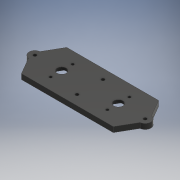
# Autodesk Inventor part: AC09
Saved by Autodesk Inventor 2017 (Build 210142000, 142)
## iProperties
Created: 2019-11-01
Part Number: AC09
Material: ABS Plastic
Document SubType Name: Modeling
Designer: Dell
Density: 1.06 g/cm^3
Appearance: Smooth - Black
Author: Dell
Autodesk Inventor part; units mm, degrees
ref_plane "YZ Plane" through (0, 0, 0) normal (1, 0, 0) x (0, 1, 0)
ref_plane "XZ Plane" through (0, 0, 0) normal (0, 1, 0) x (-1, 0, 0)
ref_plane "XY Plane" through (0, 0, 0) normal (0, 0, 1) x (1, 0, 0)
sketch "Sketch1" plane through (0, 0, 0) normal (0, 0, 1) x (1, 0, 0)
  circle A0 centre (0, 0) radius 3.5
  circle A1 centre (43.8036, 0) radius 3.5
  line L0 (-20.2073, 0) -> (-10.1036, 17.5)
  line L1 (-10.1036, 17.5) -> (10.1036, 17.5)
  line L2 (10.1036, 17.5) -> (20.2073, 0)
  line L3 (20.2073, 0) -> (10.1036, -17.5)
  line L4 (10.1036, -17.5) -> (-10.1036, -17.5)
  line L5 (-10.1036, -17.5) -> (-20.2073, 0)
  line L6 (64.0108, 0) -> (53.9072, -17.5)
  line L7 (53.9072, -17.5) -> (33.6999, -17.5)
  line L8 (33.6999, -17.5) -> (23.5963, 0)
  line L9 (23.5963, 0) -> (33.6999, 17.5)
  line L10 (33.6999, 17.5) -> (53.9072, 17.5)
  line L11 (53.9072, 17.5) -> (64.0108, 0)
  line L12 (10.1036, 17.5) -> (33.6999, 17.5)
  line L13 (10.1036, -17.5) -> (33.6999, -17.5)
  dimension "d0" = 7
  dimension "d1" = 7
  dimension "d2" = 43.8036
  dimension "d3" = 35
  constraints: 28 end point, 4 horizontal alignment, 3 coincident, 2 centre point, 2 horizontal, 26 other
  measures "d0" diameter of A0
  measures "d1" diameter of A1
  measures "d2" distance of A1.centre point (0, 0)
  measures "d3" distance between parallel lines of L4 L1
extrude "Extrusion1" add sketch "Sketch1" along normal blind 4
sketch "Sketch2" plane through (0, 0, 4) normal (0, 0, 1) x (1, 0, 0)
  circle A0 centre (43.8036, 0) radius 3.5 projected
  circle A1 centre (0, 0) radius 3.5 projected
  line L0 (-10.1036, 17.5) -> (-20.2073, 0) projected
  line L1 (-20.2073, 0) -> (-10.1036, -17.5) projected
  line L2 (53.9072, -17.5) -> (64.0108, 0) projected
  line L3 (64.0108, 0) -> (53.9072, 17.5) projected
  line L4 (57.3713, 17.5) -> (67.4749, 0)
  line L5 (67.4749, 0) -> (57.3713, -17.5)
  line L6 (-13.5677, 17.5) -> (-23.6714, 0)
  line L7 (-23.6714, 0) -> (-13.5677, -17.5)
  line L8 (53.9072, 17.5) -> (-10.1036, 17.5) projected
  line L9 (-10.1036, 17.5) -> (-13.5677, 17.5)
  line L10 (-13.5677, -17.5) -> (-10.1036, -17.5)
  line L11 (-10.1036, -17.5) -> (53.9072, -17.5) projected
  line L12 (53.9072, -17.5) -> (57.3713, -17.5)
  line L13 (64.0108, 0) -> (53.9072, 17.5) projected
  line L14 (53.9072, 17.5) -> (57.3713, 17.5)
  point P0 (-11.8357, -17.5)
  dimension "d6" = 3
  dimension "d7" = 3
  constraints: 16 end point, 4 horizontal, 2 centre point, 1 midpoint, 2 other
  measures "d6" distance between parallel lines of L3 L4
  measures "d7" distance between parallel lines of L6 L0
extrude "Extrusion2" add sketch "Sketch2" against normal up to surface (4 mm away) from surface at 0 contours L0 L1 L10 L7 L6 L9 | L14 L4 L5 L12 L2 L3
sketch "Sketch3" plane through (0, 0, 4) normal (0, 0, 1) x (1, 0, 0)
  circle A0 centre (-20.6714, 0) radius 1.25
  circle A1 centre (64.4749, 0) radius 1.25
  circle A2 centre (21.9018, 10) radius 1.25
  circle A3 centre (21.9018, -10) radius 1.25
  line L0 (21.9018, 10) -> (21.9018, -10)
  line L1 (-13.5677, 17.5) -> (57.3713, 17.5) projected
  line L2 (-20.6714, 0) -> (64.4749, 0)
  point P0 (0, 0)
  point P1 (21.9018, 17.5)
  point P2 (-10.1036, 17.5)
  point P3 (21.9018, 17.5)
  point P4 (21.9018, 0)
  dimension "d10" = 2.5
  dimension "d11" = 2.5
  dimension "d12" = 2.5
  dimension "d13" = 2.5
  dimension "d14" = 20
  dimension "d34" = 85.1463
  constraints: 4 centre point, 4 end point, 4 midpoint, 3 horizontal alignment, 1 horizontal, 1 vertical, 1 vertical alignment
  measures "d10" diameter of A0
  measures "d11" diameter of A1
  measures "d12" diameter of A2
  measures "d13" diameter of A3
  measures "d14" distance of L0.start L0.end
  measures "d34" distance of L2.end L2.start
extrude "Extrusion3" cut sketch "Sketch3" against normal through all
sketch "Sketch4" plane through (0, 0, 4) normal (0, 0, 1) x (1, 0, 0)
  line L0 (0, 8.5) -> (0, -8.5) construction
  line L1 (43.8036, 8.5) -> (43.8036, -8.5) construction
  circle A0 centre (43.8036, 0) radius 3.5 construction
  circle A1 centre (0, 0) radius 3.5 construction
  circle A2 centre (0, 8.5) radius 1.05
  circle A3 centre (0, -8.5) radius 1.05
  circle A4 centre (43.8036, -8.5) radius 1.05
  circle A5 centre (43.8036, 8.5) radius 1.05
  dimension "d19" = 17
  dimension "d20" = 17
  dimension "d21" = 2.1
  dimension "d22" = 2.1
  dimension "d23" = 2.1
  dimension "d24" = 2.1
  constraints: 8 coincident, 4 centre point, 4 end point, 2 midpoint, 2 vertical
  measures "d19" distance of L1.start L1.end
  measures "d20" distance of L0.start L0.end
  measures "d21" diameter of A2
  measures "d22" diameter of A3
  measures "d23" diameter of A4
  measures "d24" diameter of A5
extrude "Extrusion4" cut sketch "Sketch4" against normal through all
sketch "Sketch8" plane through (0, 0, 4) normal (0, 0, 1) x (1, 0, 0)
  circle A0 centre (-20.6714, 0) radius 1.25 projected
  circle A1 centre (-20.6714, 0) radius 4.4214
  circle A2 centre (64.4749, 0) radius 1.25 projected
  circle A3 centre (64.4749, 0) radius 4.4214
  point P0 (0, 0)
  dimension "d30" = 8.8427
  dimension "d31" = 8.8427
  constraints: 2 centre point, 2 coincident
  measures "d30" diameter of A1
  measures "d31" diameter of A3
extrude "Extrusion5" add sketch "Sketch8" against normal up to surface (4 mm away) from surface at 0
sketch "Sketch9" plane through (0, 0, 0) normal (0, 0, -1) x (-1, 0, 0)
  line L0 (6.3509, 0) -> (3.1754, -5.5)
  line L1 (3.1754, -5.5) -> (-3.1754, -5.5)
  line L2 (-3.1754, -5.5) -> (-6.3509, 0)
  line L3 (-6.3509, 0) -> (-3.1754, 5.5)
  line L4 (-3.1754, 5.5) -> (3.1754, 5.5)
  line L5 (3.1754, 5.5) -> (6.3509, 0)
  circle A0 centre (-43.8036, 0) radius 3.5
  line L6 (-37.4527, 0) -> (-40.6281, -5.5)
  line L7 (-40.6281, -5.5) -> (-46.979, -5.5)
  line L8 (-46.979, -5.5) -> (-50.1544, 0)
  line L9 (-50.1544, 0) -> (-46.979, 5.5)
  line L10 (-46.979, 5.5) -> (-40.6281, 5.5)
  line L11 (-40.6281, 5.5) -> (-37.4527, 0)
  circle A1 centre (-43.8036, 0) radius 3.5 projected
  circle A2 centre (0, 0) radius 3.5 projected
  dimension "d35" = 11
  dimension "d36" = 11
  constraints: 24 end point, 3 coincident, 2 horizontal alignment, 1 centre point, 26 other
  measures "d35" distance between parallel lines of L1 L4
  measures "d36" distance between parallel lines of L7 L10
extrude "Extrusion6" cut sketch "Sketch9" against normal blind 2 contours L0 L1 L2 L3 L4 L5 | A0 | L6 L7 L8 L9 L10 L11 | A2
equation "\"d7\" = d6"
equation "\"d31\" = d30"
body "Solid1"
